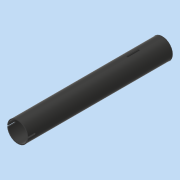
# Autodesk Inventor part: PrimaryHullLexanTube_01
Saved by Autodesk Inventor 2017 (Build 210142000, 142)
## iProperties
Created: 2016-09-09
Part Number: PrimaryHullLexanTube_01
Material: Polycarbonate, Clear
Document SubType Name: Modeling
Designer: techn
Density: 1.2 g/cm^3
Appearance: Smooth - Black
Mass: 835.743 g
Surface Area: 4410.94 cm^2
Volume: 696.452 cm^3
Author: techn
Autodesk Inventor part; units mm, degrees
ref_plane "YZ Plane" through (0, 0, 0) normal (1, 0, 0) x (0, 1, 0)
ref_plane "XY Plane" through (0, 0, 0) normal (0, 0, 1) x (1, 0, 0)
sketch "Sketch1" plane through (0, 0, 0) normal (0, 0, 1) x (1, 0, 0)
  circle A0 centre (0, 0) radius 50.8
  circle A1 centre (0, 0) radius 47.625
  dimension "d0" = 101.6
  dimension "d1" = 95.25
  constraints: 2 centre point, 2 coincident
  measures "d0" diameter of A0
  measures "d1" diameter of A1
extrude "Extrusion1" add sketch "Sketch1" along normal blind 711.2
ref_plane "Work Plane1" through (0, 50.8, 0) normal (0, 1, 0) x (-1, 0, 0)
sketch "Sketch3" plane through (0, 50.8, 0) normal (0, 1, 0) x (-1, 0, 0)
  line L0 (0, 0) -> (0, 109.855)
  line L1 (-4.7625, 109.855) -> (4.7625, 109.855)
  line L2 (4.7625, 109.855) -> (4.7625, 176.53)
  line L3 (4.7625, 176.53) -> (-4.7625, 176.53)
  line L4 (-4.7625, 176.53) -> (-4.7625, 109.855)
  dimension "d4" = 109.855
  dimension "d5" = 66.675
  dimension "d6" = 9.525
  dimension "d7" = 4.7625
  constraints: 10 end point, 2 parallel, 1 horizontal, 1 midpoint, 1 perpendicular, 1 vertical
  measures "d4" distance of L0.start L0.end
  measures "d5" distance between parallel lines of L1 L3
  measures "d6" distance between parallel lines of L2 L4
  measures "d7" distance between parallel lines of L0 L4
extrude "Extrusion2" cut sketch "Sketch3" against normal blind 25.4
fillet "Fillet1" radius 4.7625 4 edges at (-4.7625, 48.9813, 109.855) (4.7625, 48.9813, 109.855) (4.7625, 48.9813, 176.53) (-4.7625, 48.9813, 176.53)
sketch "Sketch5" plane through (0, 0, 0) normal (1, 0, 0) x (0, 1, 0)
  line L0 (50.5763, 171.7675) -> (50.5763, 114.6175) construction
  line L1 (50.5763, 114.6175) -> (50.5763, 171.7675) construction
  line L2 (50.8, 711.2) -> (-50.8, 711.2) construction
  line L3 (-50.8, 0) -> (50.8, 0) construction
  line L4 (3.175, 711.2) -> (-3.175, 711.2)
  line L5 (-3.175, 711.2) -> (-3.175, 678.7388)
  line L6 (3.175, 678.7388) -> (3.175, 711.2)
  arc A0 (-3.175, 678.7388) -> (3.175, 678.7388) centre (0, 678.7388) ccw
  line L7 (0, 769.9295) -> (0, 0) construction
  dimension "d16" = 3.175
  dimension "d17" = 32.4612
  constraints: 8 end point, 2 point on circle, 2 point on line, 2 tangent, 1 centre point, 1 horizontal, 1 parallel, 1 perpendicular, 1 vertical, 4 other
  measures "d16" radius of A0
  measures "d17" distance from line of L2 A0.centre
extrude "Extrusion4" cut sketch "Sketch5" along normal through all both and the other way through all
equation "\"d7\" = 0.5 * d6"
body "Solid1"
